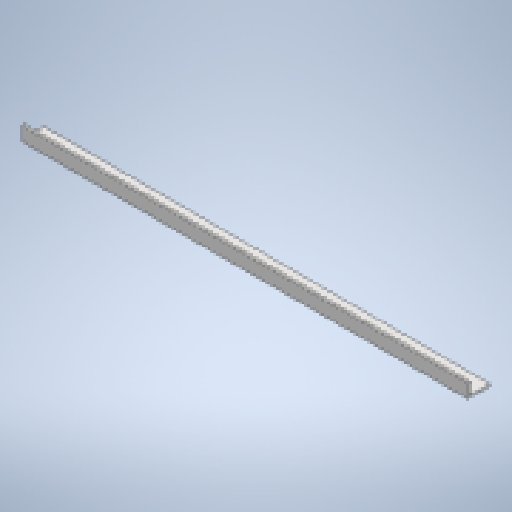
# Autodesk Inventor part: Steel_L_Bracket
Saved by Autodesk Inventor 2023 (Build 270158000, 158)
## iProperties
Created: 2022-05-01
Part Number: Steel_L_Bracket
Material: Generic
Document SubType Name: Modeling
Designer: plebbb
Density: 1 g/cm^3
Appearance: Default
Author: plebbb
Autodesk Inventor part; units mm, degrees
ref_plane "YZ Plane" through (0, 0, 0) normal (1, 0, 0) x (0, 1, 0)
ref_plane "XZ Plane" through (0, 0, 0) normal (0, 1, 0) x (-1, 0, 0)
ref_plane "XY Plane" through (0, 0, 0) normal (0, 0, 1) x (1, 0, 0)
sketch "Sketch1" plane through (0, 0, 0) normal (1, 0, 0) x (0, 1, 0)
  line L0 (0, 0) -> (0, -59.2667)
  line L1 (0, -59.2667) -> (6.35, -59.2667)
  line L2 (6.35, -59.2667) -> (6.35, -6.35)
  line L3 (6.35, -6.35) -> (38.1, -6.35)
  line L4 (38.1, -6.35) -> (38.1, 0)
  line L5 (38.1, 0) -> (0, 0)
  dimension "d0" = 38.1
  dimension "d1" = 59.2667
  dimension "d2" = 6.35
  dimension "d3" = 6.35
  constraints: 12 end point, 5 perpendicular, 1 vertical
  measures "d0" distance of L4.end L0.start
  measures "d1" distance of L0.start L0.end
  measures "d2" distance of L3.end L4.end
  measures "d3" distance of L0.end L1.end
extrude "Extrusion1" add sketch "Sketch1" along normal blind 1219.2
body "Solid1"
